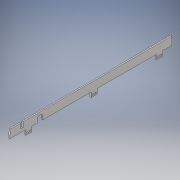
# Autodesk Inventor part: wall-inner-plunger
Saved by Autodesk Inventor 2017 (Build 210142000, 142)
## iProperties
Created: 2017-02-21
Part Number: wall-inner-plunger
Material: Generic
Document SubType Name: Modeling
Designer: John
Density: 1 g/cm^3
Appearance: Default
Author: John
Autodesk Inventor part; units mm, degrees
ref_plane "YZ Plane" through (0, 0, 0) normal (1, 0, 0) x (0, 1, 0)
ref_plane "XZ Plane" through (0, 0, 0) normal (0, 1, 0) x (-1, 0, 0)
ref_plane "XY Plane" through (0, 0, 0) normal (0, 0, 1) x (1, 0, 0)
sketch "Sketch2" plane through (0, 0, 0) normal (0, 1, 0) x (-1, 0, 0)
  line L0 (-1.5, -198.6195) -> (1.5, -198.6195)
  line L1 (1.5, -198.6195) -> (1.5, 198.6195)
  line L2 (1.5, 198.6195) -> (-1.5, 198.6195)
  line L3 (-1.5, 198.6195) -> (-1.5, -198.6195)
  line L4 (-1.5, -198.6195) -> (1.5, 198.6195) construction
  line L5 (1.5, -198.6195) -> (-1.5, 198.6195) construction
  point P0 (0, 0)
  dimension "d0" = 3
  dimension "d1" = 397.239
  constraints: 12 end point, 2 midpoint, 2 parallel, 1 horizontal, 1 perpendicular
  measures "d0" distance of L2.end L1.end
  measures "d1" distance of L1.end L0.end
extrude "Extrusion1" add sketch "Sketch2" along normal blind 20
sketch "Sketch3" plane through (1.5, 0, 198.6195) normal (1, 0, 0) x (0, 0, -1)
  line L0 (397.239, 0) -> (0, 0) projected
  line L1 (68, 0) -> (82, 0)
  line L2 (82, 0) -> (82, 7)
  line L3 (68, 7) -> (68, 0)
  arc A0 (82, 7) -> (68, 7) centre (75, 7) ccw
  arc A1 (68, 7) -> (82, 7) centre (75, 7) ccw construction
  line L4 (0, 0) -> (0, 20) projected
  point P0 (198.6195, 0)
  dimension "d4" = 14
  dimension "d5" = 7
  dimension "d6" = 14
  dimension "d9" = 75
  constraints: 6 end point, 4 point on circle, 2 centre point, 1 horizontal, 1 parallel, 1 perpendicular, 1 point on line
  measures "d4" distance of L3.start L2.end
  measures "d5" distance of L2.end L1.end
  measures "d6" diameter of A0
  measures "d9" distance from line of A0.centre L4
extrude "Extrusion2" cut sketch "Sketch3" against normal through all
sketch "Sketch4" plane through (1.5, 0, -198.6195) normal (1, 0, 0) x (0, 0, -1)
  line L0 (-329.239, 0) -> (-397.239, 0) projected
  line L1 (-397.239, 0) -> (-397.239, 20) projected
  line L2 (-397.239, 0) -> (-397.239, 20)
  line L3 (-397.239, 20) -> (-393.7125, 20)
  line L4 (-397.239, 20) -> (0, 20) projected
  line L5 (-397.239, 0) -> (-393.7125, 20)
  point P0 (-198.6195, 0)
  dimension "d10" = 10
  constraints: 6 end point, 1 point on line, 1 vertical
  measures "d10" angle of L1 L5
extrude "Extrusion3" cut sketch "Sketch4" against normal through all
sketch "Sketch6" plane through (1.5, 0, -198.6195) normal (1, 0, 0) x (0, 0, -1)
  line L0 (-393.7125, 20) -> (0, 20) projected
  line L1 (-369.839, 20) -> (-363.839, 20)
  line L2 (-363.839, 20) -> (-363.839, 8)
  line L3 (-363.839, 8) -> (-369.839, 8)
  line L4 (-369.839, 8) -> (-369.839, 20)
  line L5 (-329.239, 0) -> (-397.239, 0) construction
  line L6 (-397.239, 0) -> (-397.239, 30) construction
  point P0 (-198.6195, 0)
  dimension "d20" = 6
  dimension "d21" = 12
  dimension "d25" = 27.4
  constraints: 10 end point, 2 parallel, 1 horizontal, 1 perpendicular, 1 point on line, 1 vertical
  measures "d20" distance of L2.end L3.end
  measures "d21" distance of L1.end L2.end
  measures "d25" distance between parallel lines of L6 L4
extrude "Extrusion5" cut sketch "Sketch6" against normal blind 6
sketch "Sketch7" plane through (1.5, 0, -198.6195) normal (1, 0, 0) x (0, 0, -1)
  line L0 (-357.239, 0) -> (-342.239, 0)
  line L1 (-342.239, 0) -> (-342.239, -12)
  line L2 (-342.239, -12) -> (-357.239, -12)
  line L3 (-357.239, -12) -> (-357.239, 0)
  line L4 (-354.239, -6) -> (-345.239, -6)
  line L5 (-345.239, -6) -> (-345.239, -9)
  line L6 (-345.239, -9) -> (-354.239, -9)
  line L7 (-354.239, -9) -> (-354.239, -6)
  line L8 (-397.239, 0) -> (-329.239, 0) projected
  line L9 (-197.239, 0) -> (-182.239, 0)
  line L10 (-182.239, 0) -> (-182.239, -12)
  line L11 (-182.239, -12) -> (-197.239, -12)
  line L12 (-197.239, -12) -> (-197.239, 0)
  line L13 (-194.239, -6) -> (-185.239, -6)
  line L14 (-185.239, -6) -> (-185.239, -9)
  line L15 (-185.239, -9) -> (-194.239, -9)
  line L16 (-194.239, -9) -> (-194.239, -6)
  line L17 (-37.239, 0) -> (-22.239, 0)
  line L18 (-22.239, 0) -> (-22.239, -12)
  line L19 (-22.239, -12) -> (-37.239, -12)
  line L20 (-37.239, -12) -> (-37.239, 0)
  line L21 (-34.239, -6) -> (-25.239, -6)
  line L22 (-25.239, -6) -> (-25.239, -9)
  line L23 (-25.239, -9) -> (-34.239, -9)
  line L24 (-34.239, -9) -> (-34.239, -6)
  line L25 (-315.239, 0) -> (0, 0) projected
  point P0 (-198.6195, 0)
  dimension "d26" = 15
  dimension "d27" = 3
  dimension "d28" = 6
  dimension "d29" = 3
  dimension "d30" = 3
  dimension "d31" = 3
  dimension "d32" = 40
  dimension "d33" = 15
  dimension "d34" = 3
  dimension "d35" = 6
  dimension "d36" = 3
  dimension "d37" = 3
  dimension "d38" = 3
  dimension "d39" = 15
  dimension "d40" = 3
  dimension "d41" = 6
  dimension "d42" = 3
  dimension "d43" = 3
  dimension "d44" = 3
  dimension "d45" = 145
  dimension "d46" = 145
  constraints: 48 end point, 12 parallel, 6 horizontal, 6 perpendicular, 3 collinear
  measures "d26" distance of L1.end L2.end
  measures "d27" distance of L4.end L5.end
  measures "d28" distance between parallel lines of L0 L4
  measures "d29" distance between parallel lines of L2 L6
  measures "d30" distance between parallel lines of L3 L7
  measures "d31" distance between parallel lines of L1 L5
  measures "d32" distance from line of L3 L8.start
  measures "d33" distance of L10.end L11.end
  measures "d34" distance of L13.end L14.end
  measures "d35" distance between parallel lines of L9 L13
  measures "d36" distance between parallel lines of L11 L15
  measures "d37" distance between parallel lines of L12 L16
  measures "d38" distance between parallel lines of L10 L14
  measures "d39" distance of L18.end L19.end
  measures "d40" distance of L21.end L22.end
  measures "d41" distance between parallel lines of L17 L21
  measures "d42" distance between parallel lines of L19 L23
  measures "d43" distance between parallel lines of L20 L24
  measures "d44" distance between parallel lines of L18 L22
  measures "d45" distance between parallel lines of L1 L12
  measures "d46" distance between parallel lines of L20 L10
extrude "Extrusion6" add sketch "Sketch7" against normal blind 3
equation "\"d30\" = d29"
equation "\"d31\" = d29"
equation "\"d37\" = d36"
equation "\"d38\" = d36"
equation "\"d43\" = d42"
equation "\"d44\" = d42"
body "Solid1"
